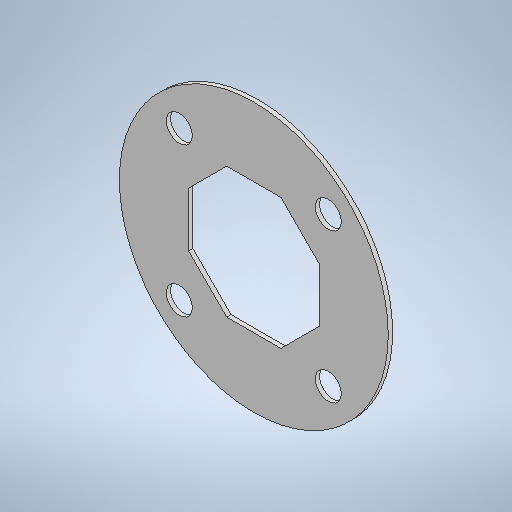
# Autodesk Inventor part: KND-0001 Flange 01
Saved by Autodesk Inventor 2026.2 (Build 302298000, 298)
## iProperties
Created: 2026-10-01
Part Number: KND-0001 Flange 01
Material: Generic
Document SubType Name: Sheet Metal
Designer: admin
Mass: 57.4544 g
Surface Area: 416.198 cm^2
Volume: 57.4544 cm^3
Density: 1 g/cm^3
Sheet Metal Rule: Default_mm
Appearance: Default
Author: admin
Autodesk Inventor part; units mm, degrees
ref_plane "YZ Plane" through (0, 0, 0) normal (1, 0, 0) x (0, 1, 0)
ref_plane "XZ Plane" through (0, 0, 0) normal (0, 1, 0) x (-1, 0, 0)
ref_plane "XY Plane" through (0, 0, 0) normal (0, 0, 1) x (1, 0, 0)
sketch "Sketch1" plane through (0, 0, 0) normal (0, 0, 1) x (1, 0, 0)
  circle A0 centre (0, 0) radius 92.5
  dimension "d0" = 185
  measures "d0" diameter of A0
extrude "Plate1" add sketch "Sketch1" along normal blind 3
sketch "Sketch2" plane through (0, 0, 3) normal (0, 0, 1) x (1, 0, 0)
  line L0 (18.6405, -45.0022) -> (45.0022, -18.6405)
  line L1 (45.0022, -18.6405) -> (45.0022, 18.6405)
  line L2 (45.0022, 18.6405) -> (18.6405, 45.0022)
  line L3 (18.6405, 45.0022) -> (-18.6405, 45.0022)
  line L4 (-18.6405, 45.0022) -> (-45.0022, 18.6405)
  line L5 (-45.0022, 18.6405) -> (-45.0022, -18.6405)
  line L6 (-45.0022, -18.6405) -> (-18.6405, -45.0022)
  line L7 (-18.6405, -45.0022) -> (18.6405, -45.0022)
  circle A0 centre (51.265, 51.265) radius 9
  circle A1 centre (-51.265, 51.265) radius 9
  circle A2 centre (-51.265, -51.265) radius 9
  circle A3 centre (51.265, -51.265) radius 9
  dimension "d2" = 18
  dimension "d3" = 18
  dimension "d4" = 18
  dimension "d5" = 18
  constraints: 16 end point, 4 centre point
  measures "d2" diameter of A0
  measures "d3" diameter of A1
  measures "d4" diameter of A2
  measures "d5" diameter of A3
extrude "Cut1" cut sketch "Sketch2" against normal blind 3
equation "\"d1\" = Thickness"
equation "\"BendRadius\" = Thickness"
equation "\"BendReliefWidth\" = Thickness"
equation "\"BendReliefDepth\" = 0.5 * Thickness"
equation "\"CornerReliefSize\" = 4 * Thickness"
equation "\"MinimumRemnant\" = 2 * Thickness"
equation "\"TransitionRadius\" = BendRadius"
equation "\"JacobiRadiusSize\" = BendRadius"
equation "\"GapSize\" = Thickness"
equation "\"Thickness\" = 3"
body "Solid1"
